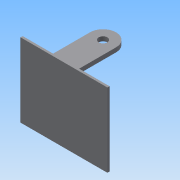
# Autodesk Inventor part: 零件3
Saved by Autodesk Inventor 2015 (Build 190159000, 159)
## iProperties
Created: 2018-04-17
Part Number: 零件3
Material: 一般
Document SubType Name: Modeling
Designer: 王博聖
Density: 1 g/cm^3
Appearance: 預設
Author: 王博聖
Autodesk Inventor part; units mm, degrees
ref_plane "YZ Plane" through (0, 0, 0) normal (1, 0, 0) x (0, 1, 0)
ref_plane "XZ Plane" through (0, 0, 0) normal (0, 1, 0) x (-1, 0, 0)
ref_plane "XY Plane" through (0, 0, 0) normal (0, 0, 1) x (1, 0, 0)
sketch "草圖1" plane through (0, 0, 0) normal (0, 0, 1) x (1, 0, 0)
  line L0 (0, 0) -> (0, -85) construction
  line L1 (-30, 0) -> (-30, -85)
  line L2 (30, -85) -> (30, 0)
  arc A0 (30, 0) -> (-30, 0) centre (0, 0) ccw
  arc A1 (-30, -85) -> (30, -85) centre (0, -85) ccw construction
  line L3 (-30, -85) -> (30, -85)
  point P0 (0, -42.5)
  dimension "d0" = 30
  dimension "d1" = 85
  constraints: 10 end point, 4 point on circle, 4 tangent, 2 centre point, 1 horizontal, 1 midpoint, 1 parallel, 1 vertical
  measures "d0" radius of A0
  measures "d1" distance from line of L0.start L3
extrude "擠出1" add sketch "草圖1" along normal blind 10
sketch "草圖2" plane through (0, 0, 0) normal (0, 0, -1) x (-1, 0, 0)
  arc A0 (30, 0) -> (-30, 0) centre (0, 0) ccw projected
  circle A1 centre (0, 0) radius 10
  dimension "d4" = 20
  constraints: 1 centre point, 1 coincident
  measures "d4" diameter of A1
extrude "擠出2" cut sketch "草圖2" against normal blind 10
sketch "草圖3" plane through (-30, -85, 0) normal (0, -1, 0) x (1, 0, 0)
  line L0 (0, 10) -> (60, 10) projected
  line L1 (-70, 10) -> (130, 10)
  line L2 (130, 10) -> (130, -160)
  line L3 (130, -160) -> (-70, -160)
  line L4 (-70, -160) -> (-70, 10)
  point P0 (30, 0)
  dimension "d7" = 100
  dimension "d8" = 200
  dimension "d9" = 170
  constraints: 8 end point, 2 parallel, 1 collinear, 1 horizontal, 1 perpendicular
  measures "d7" distance from line of point (30, 0) L2
  measures "d8" distance of L2.end L3.end
  measures "d9" distance of L3.end L1.start
extrude "擠出3" add sketch "草圖3" along normal blind 5
